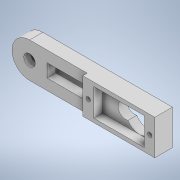
# Autodesk Inventor part: leg
Saved by Autodesk Inventor 2022 (Build 260153000, 153)
## iProperties
Created: 2021-01-08
Part Number: leg
Material: Generic
Document SubType Name: Modeling
Designer: papa
Density: 1 g/cm^3
Appearance: Default
Author: papa
Autodesk Inventor part; units mm, degrees
ref_plane "YZ Plane" through (0, 0, 0) normal (1, 0, 0) x (0, 1, 0)
ref_plane "XZ Plane" through (0, 0, 0) normal (0, 1, 0) x (-1, 0, 0)
ref_plane "XY Plane" through (0, 0, 0) normal (0, 0, 1) x (1, 0, 0)
sketch "Sketch1" plane through (0, 0, 0) normal (0, 0, 1) x (1, 0, 0)
  line L0 (8, 0) -> (67, 0)
  line L1 (67, 0) -> (67, 16)
  line L2 (67, 16) -> (8, 16)
  circle A0 centre (8, 8) radius 1.5
  circle A1 centre (56, 8) radius 6.25
  circle A2 centre (49.75, 8) radius 3.5
  arc A3 (8, 16) -> (8, 0) centre (8, 8) ccw
  point P0 (0, 0)
  point P1 (0, 8)
  point P2 (50.73, 4.64)
  point P3 (50.73, 11.36)
  dimension "d8" = 12.5
  dimension "d0" = 16
  dimension "d2" = 3
  dimension "d3" = 7
  dimension "d4" = 48
  dimension "d6" = 11
  dimension "d7" = 8
  dimension "d9" = 8
  dimension "d10" = 8
  constraints: 6 end point, 3 centre point, 3 point on circle, 1 coincident, 1 horizontal, 1 parallel, 1 perpendicular, 1 tangent, 3 other
  measures "d0" distance of L1.end L0.end
  measures "d2" diameter of A0
  measures "d3" diameter of A2
  measures "d4" distance of point (56, 8) A0.centre
  measures "d6" distance from line of L1 point (56, 8)
  measures "d7" distance from line of L0 point (56, 8)
  measures "d9" distance from line of L0 A0.centre
  measures "d10" distance from line of L0 A2.centre
extrude "Extrusion1" add sketch "Sketch1" along normal blind 8
sketch "Sketch2" plane through (0, 0, 8) normal (0, 0, 1) x (1, 0, 0)
  line L0 (62.25, 14.25) -> (39.25, 14.25)
  line L1 (39.25, 14.25) -> (39.25, 1.75)
  line L2 (39.25, 1.75) -> (62.25, 1.75)
  line L3 (62.25, 1.75) -> (62.25, 14.25)
  line L4 (67, 16) -> (8, 16) projected
  line L5 (67, 0) -> (67, 16) projected
  circle A0 centre (36.75, 8) radius 1
  circle A1 centre (64.75, 8) radius 1
  line L6 (0, 0) -> (67, 0) projected
  arc A2 (50.73, 4.64) -> (50.73, 11.36) centre (56, 8) ccw projected
  line L7 (0, 16) -> (0, 0) projected
  line L8 (0, 0) -> (34.25, 0)
  line L9 (34.25, 0) -> (34.25, 16)
  line L10 (34.25, 16) -> (0, 16)
  line L11 (0, 16) -> (0, 0)
  circle A3 centre (8, 8) radius 1.5 projected
  circle A4 centre (8, 8) radius 2.6
  line L12 (16, 5) -> (34.25, 5)
  line L13 (34.25, 5) -> (34.25, 11)
  line L14 (34.25, 11) -> (16, 11)
  line L15 (16, 11) -> (16, 5)
  dimension "d13" = 23
  dimension "d14" = 12.5
  dimension "d15" = 1.75
  dimension "d19" = 2
  dimension "d20" = 2.5
  dimension "d21" = 2.5
  dimension "d26" = 8
  dimension "d27" = 8
  dimension "d42" = 5
  dimension "d43" = 5.2
  dimension "d44" = 5
  dimension "d45" = 5
  dimension "d53" = 8
  constraints: 24 end point, 6 parallel, 3 centre point, 3 horizontal, 3 perpendicular, 1 coincident, 1 collinear, 1 point on line, 1 tangent
  measures "d13" distance of L1.end L2.end
  measures "d14" distance of L0.end L1.end
  measures "d15" distance between parallel lines of L4 L0
  measures "d19" diameter of A0
  measures "d20" distance from line of L1 A0.centre
  measures "d21" distance from line of L3 A1.centre
  measures "d26" distance from line of L6 A0.centre
  measures "d27" distance from line of L6 A1.centre
  measures "d42" distance between parallel lines of L1 L9
  measures "d43" diameter of A4
  measures "d44" distance between parallel lines of L6 L12
  measures "d45" distance between parallel lines of L14 L4
  measures "d53" distance from line of L15 A3.centre
extrude "Extrusion2" cut sketch "Sketch2" against normal blind 4 contours L3 A2 L0 | A2 L2 L1 L0 | L3 L2 A2
extrude "Extrusion6" cut sketch "Sketch2" against normal blind 2 contours L9 L14 L15 L12 L6 L7 L10 L4
extrude "Extrusion7" cut sketch "Sketch2" against normal blind 5 contours A4
extrude "Extrusion8" cut sketch "Sketch2" against normal blind 6 contours L9 L12 L15 L14
extrude "Extrusion9" cut sketch "Sketch2" against normal through all contours A0 | A1
body "Solid1"
